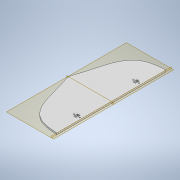
# Autodesk Inventor part: платформа_глаза
Saved by Autodesk Inventor 2020 (Build 240168000, 168)
## iProperties
Created: 2022-02-15
Part Number: платформа_глаза
Material: Типовые
Document SubType Name: Modeling
Designer: Администратор
Density: 1 g/cm^3
Appearance: По умолчанию
Author: Администратор
Autodesk Inventor part; units mm, degrees
sketch "Эскиз1" plane through (0, 0, 0) normal (0, 1, 0) x (-1, 0, 0)
  circle A0 centre (0, 0) radius 165
  line L0 (0, 165) -> (0, -165)
  dimension "d0" = 330
  constraints: 2 end point, 2 point on circle, 1 centre point, 1 coincident, 1 vertical
  measures "d0" diameter of A0
extrude "Выдавливание1" add sketch "Эскиз1" along normal blind 4 contours A0 L0 picked at (44.4959, 32.3282)
sketch "Эскиз2" plane through (0, 4, 0) normal (0, 1, 0) x (1, 0, 0)
  line L0 (0, 0) -> (-113.4659, 0)
  line L1 (0, -165) -> (0, 165) projected
  line L2 (0, -143.423) -> (-29.4077, -141.3803) construction
  line L3 (-29.4077, -141.3803) -> (-49.9234, -135.6119) construction
  line L4 (-49.9234, -135.6119) -> (-65.9786, -125.0595) construction
  line L5 (-65.9786, -125.0595) -> (-80.1797, -105.2669) construction
  line L6 (-80.1797, -105.2669) -> (-89.1079, -84.139) construction
  line L7 (-89.1079, -84.139) -> (-98.5999, -49.2669) construction
  line L8 (-98.5999, -49.2669) -> (-105.5818, -23.0172) construction
  line L9 (-105.5818, -23.0172) -> (-110.6157, -11.1357) construction
  line L10 (-110.6157, -11.1357) -> (-112.257, -3.9988) construction
  line L11 (-112.257, -3.9988) -> (-112.5892, 0) construction
  spline S0 degree 4 poles (0, -143.423) (-29.4077, -141.3803) (-49.9234, -135.6119) (-65.9786, -125.0595) (-80.1797, -105.2669) (-89.1079, -84.139) (-98.5999, -49.2669) (-105.5818, -23.0172) (-110.6157, -11.1357) (-112.257, -3.9988) (-112.5892, 0) knots 1 1 1 1 1 2 3 4 5 6 7 8 8 8 8 8
  line L12 (0, 143.423) -> (-29.4077, 141.3803) construction
  line L13 (-29.4077, 141.3803) -> (-49.9234, 135.6119) construction
  line L14 (-49.9234, 135.6119) -> (-65.9786, 125.0595) construction
  line L15 (-65.9786, 125.0595) -> (-80.1797, 105.2669) construction
  line L16 (-80.1797, 105.2669) -> (-89.1079, 84.139) construction
  line L17 (-89.1079, 84.139) -> (-98.5999, 49.2669) construction
  line L18 (-98.5999, 49.2669) -> (-105.5818, 23.0172) construction
  line L19 (-105.5818, 23.0172) -> (-110.6157, 11.1357) construction
  line L20 (-110.6157, 11.1357) -> (-112.257, 3.9988) construction
  line L21 (-112.257, 3.9988) -> (-112.5892, 0) construction
  spline S1 degree 4 poles (0, 143.423) (-29.4077, 141.3803) (-49.9234, 135.6119) (-65.9786, 125.0595) (-80.1797, 105.2669) (-89.1079, 84.139) (-98.5999, 49.2669) (-105.5818, 23.0172) (-110.6157, 11.1357) (-112.257, 3.9988) (-112.5892, 0) knots 1 1 1 1 1 2 3 4 5 6 7 8 8 8 8 8
  arc A0 (0, 165) -> (0, -165) centre (0, 0) ccw projected
  constraints: 10 symmetric about line, 2 end point, 2 point on line, 1 horizontal, 6 other
extrude "Выдавливание2" cut sketch "Эскиз2" against normal through all contours S0 L1 A0 S1
sketch "Эскиз6" plane through (0, 4, 0) normal (0, 1, 0) x (1, 0, 0)
  circle A0 centre (-5.3052, -78) radius 1.5 projected
  circle A1 centre (-20.3052, -78) radius 1.5 projected
  line L0 (-16.0562, -73) -> (-16.0562, -83) projected
  line L1 (-9.5837, -73) -> (-16.0562, -73) projected
  line L2 (-9.5837, -83) -> (-9.5837, -73) projected
  line L3 (-16.0562, -83) -> (-9.5837, -83) projected
  point P0 (0, 0)
extrude "Выдавливание6" cut sketch "Эскиз6" against normal through all
mirror "Зеркальное отражение2" about plane through (0, 0, 0) normal (0, 0, 1) of "Выдавливание6"
